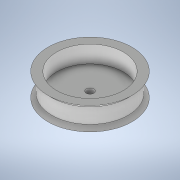
# Autodesk Inventor part: mniejsze_kolo
Saved by Autodesk Inventor 2020 (Build 240168000, 168)
## iProperties
Created: 2020-05-04
Part Number: mniejsze_kolo
Material: Generic
Document SubType Name: Modeling
Designer: Hesekiel
Density: 1 g/cm^3
Appearance: Default
Author: Hesekiel
Autodesk Inventor part; units mm, degrees
sketch "Sketch1" plane through (0, 0, 0) normal (0, 1, 0) x (-1, 0, 0)
  circle A0 centre (0, 0) radius 20
  dimension "d0" = 40
  constraints: 1 centre point, 1 coincident
  measures "d0" diameter of A0
extrude "Extrusion1" add sketch "Sketch1" along normal blind 12
sketch "Sketch2" plane through (0, 12, 0) normal (0, 1, 0) x (1, 0, 0)
  circle A0 centre (0, 0) radius 17.5
  dimension "d3" = 35
  constraints: 1 centre point, 1 coincident
  measures "d3" diameter of A0
extrude "Extrusion2" cut sketch "Sketch2" against normal blind 9
sketch "Sketch3" plane through (0, 3, 0) normal (0, 1, 0) x (1, 0, 0)
  circle A0 centre (0, 0) radius 2
  dimension "d6" = 4
  constraints: 1 centre point, 1 coincident
  measures "d6" diameter of A0
extrude "Extrusion3" cut sketch "Sketch3" against normal blind 12
sketch "Sketch4" plane through (0, 3, 0) normal (0, 1, 0) x (1, 0, 0)
  circle A0 centre (0, 0) radius 4
  circle A1 centre (0, 0) radius 2 projected
  circle A2 centre (0, 0) radius 17.5 projected
  dimension "d9" = 8
  constraints: 1 centre point, 1 coincident
  measures "d9" diameter of A0
extrude "Extrusion4" add sketch "Sketch4" along normal blind 5 contours A0
ref_plane "Work Plane1" through (0, 3, -4) normal (0, 0, 1) x (1, 0, 0)
ref_plane "Work Plane2" through (0, 3, 4) normal (0, 0, 1) x (1, 0, 0)
sketch "Sketch7" plane through (0, 3, 4) normal (0, 0, 1) x (1, 0, 0)
  line L0 (4, 5) -> (-4, 5) projected
  line L1 (-4, 0) -> (4, 0) projected
  line L2 (4, 5) -> (-4, 5) projected
  line L3 (0, 5) -> (0, 0)
  line L4 (-4, 0) -> (4, 0) projected
  circle A0 centre (0, 2.5) radius 1
  point P0 (0, -3)
  dimension "d21" = 2
  constraints: 3 midpoint, 2 end point, 1 centre point
  measures "d21" diameter of A0
extrude "Extrusion7" cut sketch "Sketch7" against normal up to surface round surface about axis through (0, 3, 0) along (0, -1, 0) radius 2 far side no
sketch "Sketch8" plane through (0, 0, 0) normal (0, -1, 0) x (1, 0, 0)
  circle A0 centre (0, 0) radius 22
  dimension "d26" = 44
  constraints: 1 centre point, 1 coincident
  measures "d26" diameter of A0
extrude "Extrusion8" add sketch "Sketch8" against normal blind 2
chamfer "Chamfer1" distance 2 angle 45 1 edges at (-22, 2, 0)
sketch "Sketch9" plane through (0, 12, 0) normal (0, 1, 0) x (1, 0, 0)
  circle A0 centre (0, 0) radius 2 projected
  circle A1 centre (0, 0) radius 22
  constraints: 1 centre point, 1 coincident
extrude "Extrusion9" add sketch "Sketch9" against normal blind 2
chamfer "Chamfer2" distance 2 angle 45 1 edges at (-22, 10, 0)
sketch "Sketch10" plane through (0, 2, 0) normal (0, 1, 0) x (1, 0, 0)
  point P0 (0, 0)
chamfer "Chamfer3" distance 0.3 angle 45 3 edges at (0.7406, 4.828, 3.9308) (0.7415, 6.1709, 3.9307) (-1, 5.4995, 3.873)
thread "Thread4" size "M2x0.4" class "6H" standard "ANSI Metric M Profile" full length
sketch "Sketch11" plane through (0, 2, 0) normal (0, 1, 0) x (1, 0, 0)
  point P0 (0, 0)
sketch "Sketch12" plane through (0, 0, 0) normal (0, -1, 0) x (1, 0, 0)
  circle A0 centre (0, 0) radius 2 projected
extrude "Extrusion10" cut sketch "Sketch12" against normal blind 3.75
ref_plane "Work Plane3" through (0, 0, 20) normal (0, 0, 1) x (1, 0, 0)
sketch "Sketch14" plane through (0, 10, 0) normal (0, -1, 0) x (1, 0, 0)
  circle A0 centre (0, 0) radius 2 projected
  circle A1 centre (0, 0) radius 17.5 projected
extrude "Extrusion12" cut sketch "Sketch14" against normal blind 12.5
sketch "Sketch15" plane through (0, 3, 0) normal (0, 1, 0) x (1, 0, 0)
  circle A0 centre (0, 0) radius 4 projected
  circle A1 centre (0, 0) radius 17.5 projected
split body "Split1" sketch "Sketch15" result two bodies curves A0 first body at (-1.7146, 5.4898, 3.0512)
move or copy body "Move Body1" bodies to move or copy 2 copy no translate (0, -8, 0)
move or copy body "Move Body2" bodies to move or copy 2 copy no rotation origin (0, 0, 0) rotation axis (1, 0, 0) rotation angle 180
move or copy body "Move Body3" bodies to move or copy 2 copy no translate (0, -8, 0)
combine bodies "Combine1" operation type add bodies to combine 3 2
sketch "Sketch16" plane through (0, 0, 0) normal (0, 1, 0) x (1, 0, 0)
  circle A0 centre (0, 0) radius 2 projected
  circle A1 centre (0, 0) radius 4 projected
extrude "Extrusion13" add sketch "Sketch16" along normal blind 3 bodies 3
sketch "Sketch17" plane through (0, -8, 0) normal (0, -1, 0) x (1, 0, 0)
  circle A0 centre (0, 0) radius 4 projected
  circle A1 centre (0, 0) radius 2 projected
  point P0 (0, 0)
extrude "Extrusion14" cut sketch "Sketch17" against normal blind 8 bodies 3
sketch "Sketch18" plane through (0, 0, 0) normal (0, -1, 0) x (1, 0, 0)
  circle A0 centre (0, 0) radius 4
  circle A1 centre (0, 0) radius 2 projected
  circle A2 centre (0, 0) radius 22 projected
  dimension "d61" = 8
  constraints: 1 centre point, 1 coincident
  measures "d61" diameter of A0
extrude "Extrusion15" add sketch "Sketch18" along normal blind 5 contours A0 bodies 3
ref_plane "Work Plane5" through (0, 0, 4) normal (0, 0, 1) x (1, 0, 0)
sketch "Sketch19" plane through (0, 0, 4) normal (0, 0, 1) x (1, 0, 0)
  line L0 (-4, -5) -> (4, -5) projected
  line L1 (4, 0) -> (-4, 0) projected
  line L2 (2, -5) -> (-2, -5) projected
  circle A0 centre (0, -2.5) radius 1.5
  point P0 (0, 0)
  dimension "d64" = 3
  constraints: 1 centre point
  measures "d64" diameter of A0
extrude "Extrusion16" cut sketch "Sketch19" against normal blind 3.5 bodies 3
thread "Thread5" size "M3x0.5" class "6H" standard "ANSI Metric M Profile" full length
body "Solid3"
